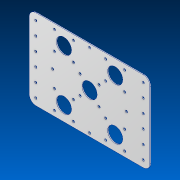
# Autodesk Inventor part: Motor Bracket Inner Panel
Saved by Autodesk Inventor 2022.2 (Build 262287000, 287)
## iProperties
Created: 2022-03-21
Part Number: Motor Bracket Inner Panel
Material: Aluminum 6061
Document SubType Name: Modeling
Designer: omard
Density: 2.7 g/cm^3
Appearance: Aluminum - Flat
Author: omard
Autodesk Inventor part; units mm, degrees
ref_plane "YZ Plane" through (0, 0, 0) normal (1, 0, 0) x (0, 1, 0)
ref_plane "XZ Plane" through (0, 0, 0) normal (0, 1, 0) x (-1, 0, 0)
ref_plane "XY Plane" through (0, 0, 0) normal (0, 0, 1) x (1, 0, 0)
derived "Motor Bracket Outer Panel.ipt"
sketch "Sketch1" plane through (0, 0, 0) normal (0, 0, 1) x (1, 0, 0)
  circle A0 centre (0, 0) radius 31.75
  line L0 (-48.4934, 48.4934) -> (48.4934, 48.4934) construction
  line L1 (48.4934, 48.4934) -> (48.4934, -48.4934) construction
  line L2 (48.4934, -48.4934) -> (-48.4934, -48.4934) construction
  line L3 (-48.4934, -48.4934) -> (-48.4934, 48.4934) construction
  line L4 (-48.4934, 48.4934) -> (48.4934, -48.4934) construction
  line L5 (48.4934, 48.4934) -> (-48.4934, -48.4934) construction
  circle A1 centre (-48.4934, 48.4934) radius 14.2875
  circle A2 centre (48.4934, 48.4934) radius 14.2875
  circle A3 centre (48.4934, -48.4934) radius 14.2875
  circle A4 centre (-48.4934, -48.4934) radius 14.2875
  line L6 (-101.6, 76.2) -> (101.6, 76.2)
  line L7 (114.3, 63.5) -> (114.3, -63.5)
  line L8 (101.6, -76.2) -> (-101.6, -76.2)
  line L9 (-114.3, -63.5) -> (-114.3, 63.5)
  line L10 (-114.3, 76.2) -> (114.3, -76.2) construction
  line L11 (114.3, 76.2) -> (-114.3, -76.2) construction
  line L12 (-101.6, -76.2) -> (-101.6, 76.2) construction
  line L13 (101.6, 76.2) -> (101.6, -76.2) construction
  arc A5 (-101.6, 76.2) -> (-114.3, 63.5) centre (-101.6, 63.5) ccw
  arc A6 (114.3, 63.5) -> (101.6, 76.2) centre (101.6, 63.5) ccw
  arc A7 (101.6, -76.2) -> (114.3, -63.5) centre (101.6, -63.5) ccw
  arc A8 (-114.3, -63.5) -> (-101.6, -76.2) centre (-101.6, -63.5) ccw
  circle A9 centre (0, 0) radius 69.85 construction
  circle A10 centre (-48.4934, 48.4934) radius 34.29 construction
  circle A11 centre (48.4934, 48.4934) radius 34.29 construction
  circle A12 centre (48.4934, -48.4934) radius 34.29 construction
  circle A13 centre (-48.4934, -48.4934) radius 34.29 construction
  line L14 (66.4539, 66.4539) -> (30.5329, 66.4539) construction
  line L15 (30.5329, 66.4539) -> (30.5329, 30.5329) construction
  line L16 (30.5329, 30.5329) -> (66.4539, 30.5329) construction
  line L17 (66.4539, 30.5329) -> (66.4539, 66.4539) construction
  line L18 (66.4539, 66.4539) -> (30.5329, 30.5329) construction
  line L19 (30.5329, 66.4539) -> (66.4539, 30.5329) construction
  line L20 (-30.5329, 66.4539) -> (-66.4539, 66.4539) construction
  line L21 (-66.4539, 66.4539) -> (-66.4539, 30.5329) construction
  line L22 (-66.4539, 30.5329) -> (-30.5329, 30.5329) construction
  line L23 (-30.5329, 30.5329) -> (-30.5329, 66.4539) construction
  line L24 (-30.5329, 66.4539) -> (-66.4539, 30.5329) construction
  line L25 (-66.4539, 66.4539) -> (-30.5329, 30.5329) construction
  line L26 (-30.5329, -30.5329) -> (-66.4539, -30.5329) construction
  line L27 (-66.4539, -30.5329) -> (-66.4539, -66.4539) construction
  line L28 (-66.4539, -66.4539) -> (-30.5329, -66.4539) construction
  line L29 (-30.5329, -66.4539) -> (-30.5329, -30.5329) construction
  line L30 (-30.5329, -30.5329) -> (-66.4539, -66.4539) construction
  line L31 (-66.4539, -30.5329) -> (-30.5329, -66.4539) construction
  line L32 (66.4539, -30.5329) -> (30.5329, -30.5329) construction
  line L33 (30.5329, -30.5329) -> (30.5329, -66.4539) construction
  line L34 (30.5329, -66.4539) -> (66.4539, -66.4539) construction
  line L35 (66.4539, -66.4539) -> (66.4539, -30.5329) construction
  line L36 (66.4539, -30.5329) -> (30.5329, -66.4539) construction
  line L37 (30.5329, -30.5329) -> (66.4539, -66.4539) construction
  line L38 (-17.9605, 17.9605) -> (17.9605, 17.9605) construction
  line L39 (17.9605, 17.9605) -> (17.9605, -17.9605) construction
  line L40 (17.9605, -17.9605) -> (-17.9605, -17.9605) construction
  line L41 (-17.9605, -17.9605) -> (-17.9605, 17.9605) construction
  line L42 (-17.9605, 17.9605) -> (17.9605, -17.9605) construction
  line L43 (17.9605, 17.9605) -> (-17.9605, -17.9605) construction
  circle A14 centre (0, 0) radius 14.2875
  point P0 (101.6, -38.1)
  point P1 (101.6, 38.1)
  point P2 (-101.6, 38.1)
  point P3 (-101.6, -38.1)
  point P4 (-101.6, 63.5)
  point P5 (-101.6, -63.5)
  point P6 (101.6, -63.5)
  point P7 (101.6, 63.5)
  point P8 (-101.6, 12.7)
  point P9 (-101.6, -12.7)
  point P10 (101.6, 12.7)
  point P11 (101.6, -12.7)
  point P12 (0, 69.85)
  point P13 (69.85, 0)
  point P14 (0, -69.85)
  point P15 (-69.85, 0)
extrude "Extrusion1" add sketch "Sketch1" along normal blind 1.6256 contours A0 | L6 A6 L7 A7 L8 A8 L9 A5
hole "Hole1" at (101.6, -38.1, 0) at (101.6, 38.1, 0) at (-101.6, 38.1, 0) at (-101.6, -38.1, 0) at (-101.6, 63.5, 0) at (-101.6, -63.5, 0) at (101.6, -63.5, 0) at (101.6, 63.5, 0) at (-101.6, 12.7, 0) at (-101.6, -12.7, 0) at (101.6, 12.7, 0) at (101.6, -12.7, 0) at (0, 69.85, 0) at (69.85, 0, 0) at (0, -69.85, 0) at (-69.85, 0, 0) at (66.4539, 66.4539, 0) at (30.5329, 66.4539, 0) at (30.5329, 30.5329, 0) at (66.4539, 30.5329, 0) at (-66.4539, 66.4539, 0) at (-66.4539, 30.5329, 0) at (-30.5329, 30.5329, 0) at (-30.5329, 66.4539, 0) at (-30.5329, -30.5329, 0) at (-66.4539, -30.5329, 0) at (-66.4539, -66.4539, 0) at (-30.5329, -66.4539, 0) at (66.4539, -30.5329, 0) at (30.5329, -30.5329, 0) at (30.5329, -66.4539, 0) at (66.4539, -66.4539, 0) at (17.9605, 17.9605, 0) at (-17.9605, 17.9605, 0) at (-17.9605, -17.9605, 0) at (17.9605, -17.9605, 0) direction (0, 0, 1) diameter 4.318 end through all start extended yes
body "Solid2"
